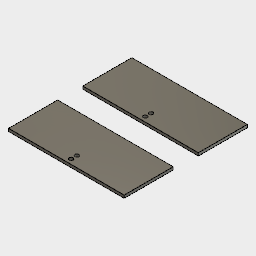
Box Flap v5 (Autodesk Fusion 360 design; units mm, degrees)
Autodesk Fusion 360 part; units mm, degrees
sketch "Sketch1" plane through (0, 0, 0) normal (0, 1, 0) x (1, 0, 0)
  line L0 (0, 0) -> (-120, 0)
  line L1 (-120, 0) -> (-120, 51)
  line L2 (-120, 51) -> (0, 51)
  line L3 (0, 51) -> (0, 0)
  line L4 (0.4421, 127.4826) -> (-119.5579, 127.4826)
  line L5 (-119.5579, 127.4826) -> (-119.5579, 76.4826)
  line L6 (-119.5579, 76.4826) -> (0.4421, 76.4826)
  line L7 (0.4421, 76.4826) -> (0.4421, 127.4826)
  circle A0 centre (-60, 5) radius 2
  circle A1 centre (-60, 11) radius 2
  circle A2 centre (-59.5579, 87.4826) radius 2
  circle A3 centre (-59.5579, 81.4826) radius 2
  dimension "d1" = 120
  dimension "d2" = 51
  dimension "d3" = 51
  dimension "d6" = 4
  dimension "d7" = 4
  dimension "d12" = 4
  dimension "d13" = 4
  dimension "d14" = 5
  dimension "d15" = 6
  dimension "d16" = 5
  dimension "d17" = 6
  constraint horizontal L0
  constraint vertical L1
  constraint horizontal L2
  constraint vertical L3
  constraint horizontal L4
  constraint vertical L5
  constraint horizontal L6
  constraint vertical L7
  constraint midpoint L6
  constraint midpoint L0
  measures "d6" diameter of A0
  measures "d7" diameter of A1
  measures "d12" diameter of A3
  measures "d13" diameter of A2
extrude "Extrude2" add sketch "Sketch1" along normal blind 3 makes body 1 at (-60.0498, 0, -38.3315) makes body 2 at (-59.6078, 0, -114.8141)
extrude "Extrude1" [suppressed]
